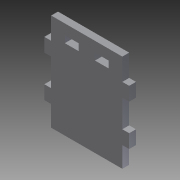
# Autodesk Inventor part: support
Saved by Autodesk Inventor 2011 (Build 150239000, 239)
## iProperties
Created: 2011-02-21
Part Number: support
Document SubType Name: Modeling
Designer: adowning
Density: 1 g/cm^3
Author: adowning
Autodesk Inventor part; units mm, degrees
ref_plane "YZ Plane" through (0, 0, 0) normal (1, 0, 0) x (0, 1, 0)
ref_plane "XZ Plane" through (0, 0, 0) normal (0, 1, 0) x (-1, 0, 0)
ref_plane "XY Plane" through (0, 0, 0) normal (0, 0, 1) x (1, 0, 0)
sketch "Sketch1" plane through (0, 0, 0) normal (0, 0, 1) x (1, 0, 0)
  line L0 (-16.9002, 13.704) -> (49.1398, 13.704)
  line L1 (49.1398, 13.704) -> (49.1398, -76.466)
  line L2 (-16.9002, 13.704) -> (-16.9002, -76.466)
  line L3 (-16.9002, -76.466) -> (49.1398, -76.466)
  line L4 (49.1398, -76.466) -> (49.1398, -57.416)
  line L5 (49.1398, -57.416) -> (55.4898, -57.416)
  line L6 (55.4898, -57.416) -> (55.4898, -44.716)
  line L7 (55.4898, -44.716) -> (49.1398, -44.716)
  line L8 (49.1398, -44.716) -> (49.1398, -19.316)
  line L9 (49.1398, -19.316) -> (55.4898, -19.316)
  line L10 (55.4898, -19.316) -> (55.4898, -6.616)
  line L11 (55.4898, -6.616) -> (49.1398, -6.616)
  line L12 (-16.9002, -76.466) -> (-16.9002, -57.416)
  line L13 (-16.9002, -57.416) -> (-23.2502, -57.416)
  line L14 (-23.2502, -57.416) -> (-23.2502, -44.716)
  line L15 (-23.2502, -44.716) -> (-16.9002, -44.716)
  line L16 (-16.9002, -44.716) -> (-16.9002, -19.316)
  line L17 (-16.9002, -19.316) -> (-23.2502, -19.316)
  line L18 (-23.2502, -19.316) -> (-23.2502, -6.616)
  line L19 (-23.2502, -6.616) -> (-16.9002, -6.616)
  point P0 (0, 0)
  dimension "d0" = 66.04
  dimension "d1" = 90.17
  dimension "d2" = 90.17
  dimension "d3" = 19.05
  dimension "d4" = 6.35
  dimension "d5" = 12.7
  dimension "d6" = 25.4
  dimension "d7" = 6.35
  dimension "d8" = 12.7
  dimension "d9" = 19.05
  dimension "d10" = 6.35
  dimension "d11" = 12.7
  dimension "d12" = 25.4
  dimension "d13" = 12.7
  constraints: 40 end point, 10 perpendicular, 8 point on line, 4 parallel, 1 horizontal
  measures "d0" distance of L0.start L0.end
  measures "d1" distance of L0.end L1.end
  measures "d2" distance of L0.start L2.end
  measures "d3" distance of L1.end L4.end
  measures "d4" distance of L4.end L5.end
  measures "d5" distance of L5.end L6.end
  measures "d6" distance of L7.end L8.end
  measures "d7" distance of L8.end L9.end
  measures "d8" distance of L9.end L10.end
  measures "d9" distance of L2.end L12.end
  measures "d10" distance of L12.end L13.end
  measures "d11" distance of L13.end L14.end
  measures "d12" distance of L15.end L16.end
  measures "d13" distance of L17.end L18.end
extrude "Extrusion1" add sketch "Sketch1" along normal blind 6.35
sketch "Sketch2" plane through (0, 0, 6.35) normal (0, 0, 1) x (1, 0, 0)
  line L0 (-16.9002, 13.704) -> (49.1398, 13.704) projected
  line L1 (-16.9002, 13.704) -> (-4.2002, 13.704)
  line L2 (-4.2002, 13.704) -> (-4.2002, 4.179)
  line L3 (-4.2002, 4.179) -> (8.4998, 4.179)
  line L4 (8.4998, 4.179) -> (8.4998, -2.171)
  line L5 (8.4998, -2.171) -> (-4.2002, -2.171)
  line L6 (-4.2002, -2.171) -> (-4.2002, 4.179)
  line L7 (49.1398, 13.704) -> (36.4398, 13.704)
  line L8 (36.4398, 13.704) -> (36.4398, 4.179)
  line L9 (36.4398, 4.179) -> (23.7398, 4.179)
  line L10 (23.7398, 4.179) -> (23.7398, -2.171)
  line L11 (23.7398, -2.171) -> (36.4398, -2.171)
  line L12 (36.4398, -2.171) -> (36.4398, 4.179)
  point P0 (0, 0)
  dimension "d16" = 12.7
  dimension "d17" = 9.525
  dimension "d18" = 12.7
  dimension "d19" = 6.35
  dimension "d20" = 12.7
  dimension "d21" = 12.7
  constraints: 24 end point, 6 perpendicular, 4 parallel, 2 point on line
  measures "d16" distance of L0.start L1.end
  measures "d17" distance of L1.end L2.end
  measures "d18" distance of L2.end L3.end
  measures "d19" distance of L3.end L4.end
  measures "d20" distance of L0.end L7.end
  measures "d21" distance of L8.end L9.end
extrude "Extrusion2" cut sketch "Sketch2" against normal blind 25.4
body "Solid1"
